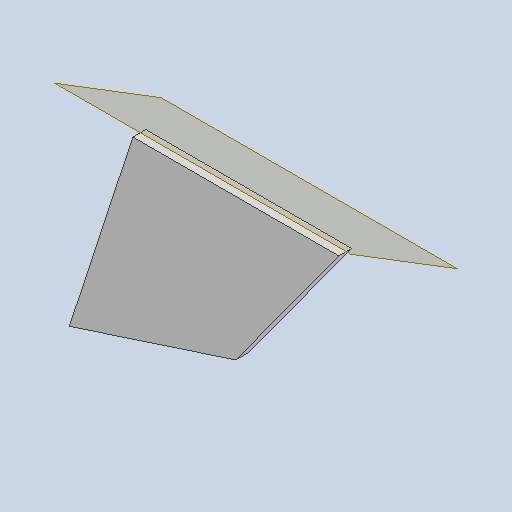
# Autodesk Inventor part: Pieza5
Saved by Autodesk Inventor 2024 (Build 280153000, 153)
## iProperties
Created: 2025-08-12
Part Number: Pieza5
Material: Genérico
Document SubType Name: Modeling
Designer: sergi
Density: 1 g/cm^3
Appearance: Valor por defecto
Author: sergi
Autodesk Inventor part; units mm, degrees
ref_plane "YZ Plane" through (0, 0, 0) normal (1, 0, 0) x (0, 1, 0)
ref_plane "XZ Plane" through (0, 0, 0) normal (0, 1, 0) x (-1, 0, 0)
ref_plane "XY Plane" through (0, 0, 0) normal (0, 0, 1) x (1, 0, 0)
sketch "Boceto1" plane through (0, 0, 0) normal (0, 0, 1) x (1, 0, 0)
  line L0 (-5.1008, 7.9792) -> (-5.1008, 9.0792) projected
  line L1 (-5.1008, 9.0792) -> (-5.9, 9.0792) projected
  line L2 (-5.1008, 7.9792) -> (-5.9, 9.0792) projected
  line L3 (-6.147, 8.3191) -> (-5.1008, 7.9792) projected
  line L4 (-5.1008, 7.9792) -> (-5.9, 9.0792) projected
  line L5 (-6.147, 8.3191) -> (-5.9, 9.0792) projected
  line L6 (-6.147, 8.3191) -> (-5.9, 9.0792)
  line L7 (-5.1008, 9.0792) -> (-5.9, 9.0792)
  line L8 (-5.1008, 7.9792) -> (-5.1008, 9.0792)
  line L9 (-5.1008, 7.9792) -> (-5.9, 9.0792)
  line L10 (-5.1008, 7.9792) -> (-6.147, 8.3191)
  line L11 (-6.147, 8.3191) -> (-6.3939, 7.559)
  line L12 (-6.3939, 7.559) -> (-5.1008, 7.9792)
  line L13 (-5.1008, 9.0792) -> (-4.3016, 9.0792)
  line L14 (-5.1008, 7.9792) -> (-4.3016, 9.0792)
  point P0 (0, 0)
  constraints: 18 end point, 8 collinear, 1 perpendicular
extrude "Extrusión1" add sketch "Boceto1" along normal blind 0.1
ref_plane "Plano de trabajo1" through (-4.3016, 9.0792, 0) normal (0, 0.8507, -0.5257) x (-1, 0, 0)
